Autodesk Inventor part; units mm, degrees
(part 2 of 2)
sketch "Sketch20" plane through (0, 0, 0) normal (0, 0, -1) x (-1, 0, 0)
  circle A0 centre (71.2839, 4.1003) radius 2.05 projected
  line L0 (18.7922, 50.612) -> (16.144, 53.2617) projected
  line L1 (16.144, 53.2617) -> (8.7758, 73.5057) projected
  line L2 (8.7758, 73.5057) -> (-5.3196, 68.3754) projected
  line L3 (-5.3196, 68.3754) -> (-0.5189, 55.1856) projected
  line L4 (-0.5189, 55.1856) -> (-4.7023, 50.8809) projected
  line L5 (-4.7023, 50.8809) -> (-16.3483, 60.653) projected
  line L6 (-16.3483, 60.653) -> (-25.9901, 49.1624) projected
  line L7 (-25.9901, 49.1624) -> (-15.1841, 40.095) projected
  line L8 (-15.1841, 40.095) -> (-24.8028, 30.1972) projected
  line L9 (-24.8028, 30.1972) -> (-34.8028, 30.1972) projected
  line L10 (-34.8028, 30.1972) -> (-34.8028, 10.1972) projected
  line L11 (-34.8028, 10.1972) -> (-29.0502, 10.1972) projected
  arc A1 (-25.3547, 7.7279) -> (-29.0502, 10.1972) centre (-29.0502, 6.1972) ccw projected
  line L12 (-25.3547, 7.7279) -> (-20.83, -3.1958) projected
  arc A2 (-21.6971, -7.5549) -> (-20.83, -3.1958) centre (-24.5255, -4.7265) ccw projected
  line L13 (-21.6971, -7.5549) -> (-25.7648, -11.6226) projected
  line L14 (-25.7648, -11.6226) -> (-11.6226, -25.7648) projected
  line L15 (-11.6226, -25.7648) -> (-7.5549, -21.6971) projected
  arc A3 (-3.1958, -20.83) -> (-7.5549, -21.6971) centre (-4.7265, -24.5255) ccw projected
  line L16 (-3.1958, -20.83) -> (7.7279, -25.3547) projected
  arc A4 (10.1972, -29.0502) -> (7.7279, -25.3547) centre (6.1972, -29.0502) ccw projected
  line L17 (10.1972, -29.0502) -> (10.1972, -34.8028) projected
  line L18 (10.1972, -34.8028) -> (30.1972, -34.8028) projected
  line L19 (30.1972, -34.8028) -> (30.1972, -28.1837) projected
  arc A5 (32.6218, -22.4466) -> (30.1972, -28.1837) centre (38.1972, -28.1837) ccw projected
  line L20 (32.6218, -22.4466) -> (53.0032, -2.6398) projected
  arc A6 (60.0735, -2.7409) -> (53.0032, -2.6398) centre (56.4878, -6.2256) ccw projected
  line L21 (60.0735, -2.7409) -> (62.5248, -5.2633) projected
  line L22 (62.5248, -5.2633) -> (77.9523, 0.8165) projected
  line L23 (77.9523, 0.8165) -> (73.9192, 11.0505) projected
  line L24 (73.9192, 11.0505) -> (50.612, 18.7922) projected
  line L25 (50.612, 18.7922) -> (36.1071, 4.2873) projected
  arc A7 (4.2873, 36.1071) -> (36.1071, 4.2873) centre (20.1972, 20.1972) ccw projected
  line L26 (4.2873, 36.1071) -> (18.7922, 50.612) projected
  circle A8 centre (2.0841, -7.6945) radius 2.075 projected
  circle A9 centre (-7.6945, 2.0841) radius 2.075 projected
  circle A10 centre (14.9946, -12.6504) radius 2.075 projected
  circle A11 centre (-12.6504, 14.9946) radius 2.075 projected
  line L27 (-18.8014, 27.6377) -> (-12.6669, 23.6539) projected
  arc A12 (-12.8482, 20.1946) -> (-12.6669, 23.6539) centre (-13.7562, 21.9766) ccw projected
  line L28 (-12.8482, 20.1946) -> (-19.3655, 16.8739) projected
  arc A13 (-22.272, 18.5798) -> (-19.3655, 16.8739) centre (-20.2735, 18.6559) ccw projected
  arc A14 (-21.8703, 26.245) -> (-22.272, 18.5798) centre (20.1972, 20.1972) ccw projected
  arc A15 (-18.8014, 27.6377) -> (-21.8703, 26.245) centre (-19.8907, 25.9604) ccw projected
  line L29 (-18.4561, 11.1323) -> (-11.2317, 9.988) projected
  arc A16 (-9.9903, 6.754) -> (-11.2317, 9.988) centre (-11.5446, 8.0127) ccw projected
  line L30 (-9.9903, 6.754) -> (-14.5934, 1.0696) projected
  arc A17 (-17.9425, 1.4458) -> (-14.5934, 1.0696) centre (-16.1477, 2.3282) ccw projected
  arc A18 (-20.6932, 8.6117) -> (-17.9425, 1.4458) centre (20.1972, 20.1972) ccw projected
  arc A19 (-18.4561, 11.1323) -> (-20.6932, 8.6117) centre (-18.769, 9.1569) ccw projected
  line L31 (16.8739, -19.3655) -> (20.1946, -12.8482) projected
  arc A20 (23.6539, -12.6669) -> (20.1946, -12.8482) centre (21.9766, -13.7562) ccw projected
  line L32 (23.6539, -12.6669) -> (27.6377, -18.8014) projected
  arc A21 (26.245, -21.8703) -> (27.6377, -18.8014) centre (25.9604, -19.8907) ccw projected
  arc A22 (18.5798, -22.272) -> (26.245, -21.8703) centre (20.1972, 20.1972) ccw projected
  arc A23 (16.8739, -19.3655) -> (18.5798, -22.272) centre (18.6559, -20.2735) ccw projected
  line L33 (1.0696, -14.5934) -> (6.754, -9.9903) projected
  arc A24 (9.988, -11.2317) -> (6.754, -9.9903) centre (8.0127, -11.5446) ccw projected
  line L34 (9.988, -11.2317) -> (11.1323, -18.4561) projected
  arc A25 (8.6117, -20.6932) -> (11.1323, -18.4561) centre (9.1569, -18.769) ccw projected
  arc A26 (1.4458, -17.9425) -> (8.6117, -20.6932) centre (20.1972, 20.1972) ccw projected
  arc A27 (1.0696, -14.5934) -> (1.4458, -17.9425) centre (2.3282, -16.1477) ccw projected
  line L35 (-11.4273, -3.8057) -> (-4.3621, -1.9126) projected
  arc A28 (-1.9126, -4.3621) -> (-4.3621, -1.9126) centre (-3.8444, -3.8444) ccw projected
  line L36 (-1.9126, -4.3621) -> (-3.8057, -11.4273) projected
  arc A29 (-7.0183, -12.4458) -> (-3.8057, -11.4273) centre (-5.7376, -10.9097) ccw projected
  arc A30 (-12.4458, -7.0183) -> (-7.0183, -12.4458) centre (20.1972, 20.1972) ccw projected
  arc A31 (-11.4273, -3.8057) -> (-12.4458, -7.0183) centre (-10.9097, -5.7376) ccw projected
  circle A32 centre (38.4172, 1.8124) radius 1.5 projected
  circle A33 centre (1.8124, 1.8124) radius 1.5 projected
  circle A34 centre (1.8124, 38.4172) radius 1.5 projected
  circle A35 centre (26.1972, -31.0318) radius 1.5 projected
  circle A36 centre (-31.0318, 14.1972) radius 1.5 projected
  circle A37 centre (-31.0318, 26.1972) radius 1.5 projected
  circle A38 centre (14.1972, -31.0318) radius 1.5 projected
  circle A39 centre (-11.7845, -20.2698) radius 1.5 projected
  circle A40 centre (-20.2698, -11.7845) radius 1.5 projected
  circle A41 centre (6.2141, 68.8487) radius 2 projected
  circle A42 centre (-0.3638, 66.4546) radius 2 projected
  circle A43 centre (-18.4881, 52.658) radius 2 projected
  point P0 (0, 0)
hole "Hole4" at (-6.2141, 68.8487, 0) at (0.3638, 66.4546, 0) at (18.4881, 52.658, 0) direction (0, 0, 1) diameter 3 depth 17
fillet "Fillet9" radius 6 1 edges at (24.8028, 30.1972, 2.5)
fillet "Fillet10" radius 3 2 edges at (15.1841, 40.095, 2.5) (4.7023, 50.8809, 2.5)
fillet "Fillet11" radius 4 1 edges at (0.5189, 55.1856, 2.5)
fillet "Fillet12" radius 8 1 edges at (-16.144, 53.2617, 2.5)
sketch "Sketch21" plane through (0, 0, 0) normal (0, 0, -1) x (-1, 0, 0)
  circle A0 centre (-0.3638, 66.4546) radius 1.5 projected
  circle A1 centre (6.2141, 68.8487) radius 1.5 projected
  circle A2 centre (-18.4881, 52.658) radius 1.5 projected
  circle A3 centre (71.2839, 4.1003) radius 2.05 projected
  line L0 (18.7922, 50.612) -> (17.3969, 52.0081) projected
  arc A4 (15.5379, 54.9271) -> (17.3969, 52.0081) centre (23.0554, 57.6633) ccw projected
  line L1 (15.5379, 54.9271) -> (8.7758, 73.5057) projected
  line L2 (8.7758, 73.5057) -> (-5.3196, 68.3754) projected
  line L3 (-5.3196, 68.3754) -> (-1.3768, 57.5426) projected
  arc A5 (-2.267, 53.3868) -> (-1.3768, 57.5426) centre (-5.1356, 56.1745) ccw projected
  line L4 (-2.267, 53.3868) -> (-2.7588, 52.8808) projected
  arc A6 (-6.8386, 52.6734) -> (-2.7588, 52.8808) centre (-4.9102, 54.9716) ccw projected
  line L5 (-6.8386, 52.6734) -> (-16.3483, 60.653) projected
  line L6 (-16.3483, 60.653) -> (-25.9901, 49.1624) projected
  line L7 (-25.9901, 49.1624) -> (-17.6563, 42.1695) projected
  arc A7 (-17.4332, 37.7806) -> (-17.6563, 42.1695) centre (-19.5847, 39.8713) ccw projected
  line L8 (-17.4332, 37.7806) -> (-23.0356, 32.0156) projected
  arc A8 (-27.3385, 30.1972) -> (-23.0356, 32.0156) centre (-27.3385, 36.1972) ccw projected
  line L9 (-27.3385, 30.1972) -> (-34.8028, 30.1972) projected
  line L10 (-34.8028, 30.1972) -> (-34.8028, 10.1972) projected
  line L11 (-34.8028, 10.1972) -> (-29.0502, 10.1972) projected
  arc A9 (-25.3547, 7.7279) -> (-29.0502, 10.1972) centre (-29.0502, 6.1972) ccw projected
  line L12 (-25.3547, 7.7279) -> (-20.83, -3.1958) projected
  arc A10 (-21.6971, -7.5549) -> (-20.83, -3.1958) centre (-24.5255, -4.7265) ccw projected
  line L13 (-21.6971, -7.5549) -> (-25.7648, -11.6226) projected
  line L14 (-25.7648, -11.6226) -> (-11.6226, -25.7648) projected
  line L15 (-11.6226, -25.7648) -> (-7.5549, -21.6971) projected
  arc A11 (-3.1958, -20.83) -> (-7.5549, -21.6971) centre (-4.7265, -24.5255) ccw projected
  line L16 (-3.1958, -20.83) -> (7.7279, -25.3547) projected
  arc A12 (10.1972, -29.0502) -> (7.7279, -25.3547) centre (6.1972, -29.0502) ccw projected
  line L17 (10.1972, -29.0502) -> (10.1972, -34.8028) projected
  line L18 (10.1972, -34.8028) -> (30.1972, -34.8028) projected
  line L19 (30.1972, -34.8028) -> (30.1972, -28.1837) projected
  arc A13 (32.6218, -22.4466) -> (30.1972, -28.1837) centre (38.1972, -28.1837) ccw projected
  line L20 (32.6218, -22.4466) -> (53.0032, -2.6398) projected
  arc A14 (60.0735, -2.7409) -> (53.0032, -2.6398) centre (56.4878, -6.2256) ccw projected
  line L21 (60.0735, -2.7409) -> (62.5248, -5.2633) projected
  line L22 (62.5248, -5.2633) -> (77.9523, 0.8165) projected
  line L23 (77.9523, 0.8165) -> (73.9192, 11.0505) projected
  line L24 (73.9192, 11.0505) -> (50.612, 18.7922) projected
  line L25 (50.612, 18.7922) -> (36.1071, 4.2873) projected
  arc A15 (4.2873, 36.1071) -> (36.1071, 4.2873) centre (20.1972, 20.1972) ccw projected
  line L26 (4.2873, 36.1071) -> (18.7922, 50.612) projected
  circle A16 centre (2.0841, -7.6945) radius 2.075 projected
  circle A17 centre (-7.6945, 2.0841) radius 2.075 projected
  circle A18 centre (14.9946, -12.6504) radius 2.075 projected
  circle A19 centre (-12.6504, 14.9946) radius 2.075 projected
  line L27 (-18.8014, 27.6377) -> (-12.6669, 23.6539) projected
  arc A20 (-12.8482, 20.1946) -> (-12.6669, 23.6539) centre (-13.7562, 21.9766) ccw projected
  line L28 (-12.8482, 20.1946) -> (-19.3655, 16.8739) projected
  arc A21 (-22.272, 18.5798) -> (-19.3655, 16.8739) centre (-20.2735, 18.6559) ccw projected
  arc A22 (-21.8703, 26.245) -> (-22.272, 18.5798) centre (20.1972, 20.1972) ccw projected
  arc A23 (-18.8014, 27.6377) -> (-21.8703, 26.245) centre (-19.8907, 25.9604) ccw projected
  line L29 (-18.4561, 11.1323) -> (-11.2317, 9.988) projected
  arc A24 (-9.9903, 6.754) -> (-11.2317, 9.988) centre (-11.5446, 8.0127) ccw projected
  line L30 (-9.9903, 6.754) -> (-14.5934, 1.0696) projected
  arc A25 (-17.9425, 1.4458) -> (-14.5934, 1.0696) centre (-16.1477, 2.3282) ccw projected
  arc A26 (-20.6932, 8.6117) -> (-17.9425, 1.4458) centre (20.1972, 20.1972) ccw projected
  arc A27 (-18.4561, 11.1323) -> (-20.6932, 8.6117) centre (-18.769, 9.1569) ccw projected
  line L31 (16.8739, -19.3655) -> (20.1946, -12.8482) projected
  arc A28 (23.6539, -12.6669) -> (20.1946, -12.8482) centre (21.9766, -13.7562) ccw projected
  line L32 (23.6539, -12.6669) -> (27.6377, -18.8014) projected
  arc A29 (26.245, -21.8703) -> (27.6377, -18.8014) centre (25.9604, -19.8907) ccw projected
  arc A30 (18.5798, -22.272) -> (26.245, -21.8703) centre (20.1972, 20.1972) ccw projected
  arc A31 (16.8739, -19.3655) -> (18.5798, -22.272) centre (18.6559, -20.2735) ccw projected
  line L33 (1.0696, -14.5934) -> (6.754, -9.9903) projected
  arc A32 (9.988, -11.2317) -> (6.754, -9.9903) centre (8.0127, -11.5446) ccw projected
  line L34 (9.988, -11.2317) -> (11.1323, -18.4561) projected
  arc A33 (8.6117, -20.6932) -> (11.1323, -18.4561) centre (9.1569, -18.769) ccw projected
  arc A34 (1.4458, -17.9425) -> (8.6117, -20.6932) centre (20.1972, 20.1972) ccw projected
  arc A35 (1.0696, -14.5934) -> (1.4458, -17.9425) centre (2.3282, -16.1477) ccw projected
  line L35 (-11.4273, -3.8057) -> (-4.3621, -1.9126) projected
  arc A36 (-1.9126, -4.3621) -> (-4.3621, -1.9126) centre (-3.8444, -3.8444) ccw projected
  line L36 (-1.9126, -4.3621) -> (-3.8057, -11.4273) projected
  arc A37 (-7.0183, -12.4458) -> (-3.8057, -11.4273) centre (-5.7376, -10.9097) ccw projected
  arc A38 (-12.4458, -7.0183) -> (-7.0183, -12.4458) centre (20.1972, 20.1972) ccw projected
  arc A39 (-11.4273, -3.8057) -> (-12.4458, -7.0183) centre (-10.9097, -5.7376) ccw projected
  circle A40 centre (38.4172, 1.8124) radius 1.5 projected
  circle A41 centre (1.8124, 1.8124) radius 1.5 projected
  circle A42 centre (1.8124, 38.4172) radius 1.5 projected
  circle A43 centre (26.1972, -31.0318) radius 1.5 projected
  circle A44 centre (-31.0318, 14.1972) radius 1.5 projected
  circle A45 centre (-31.0318, 26.1972) radius 1.5 projected
  circle A46 centre (14.1972, -31.0318) radius 1.5 projected
  circle A47 centre (-11.7845, -20.2698) radius 1.5 projected
  circle A48 centre (-20.2698, -11.7845) radius 1.5 projected
  line L37 (31.6767, -17.1814) -> (25.3462, -7.4334)
  line L38 (25.3462, -7.4334) -> (41.5924, -1.0919)
  line L39 (41.5924, -1.0919) -> (43.4186, -5.7705)
  line L40 (43.4186, -5.7705) -> (31.6767, -17.1814)
  line L41 (23.6539, -12.6669) -> (27.6377, -18.8014) projected
  line L42 (46.5296, -1.8774) -> (43.6875, 5.5512)
  line L43 (43.6875, 5.5512) -> (51.5169, 13.3805)
  line L44 (51.5169, 13.3805) -> (46.5296, -1.8774)
  line L45 (52.3971, 3.0674) -> (55.3518, 12.1067)
  line L46 (55.3518, 12.1067) -> (66.1951, 8.505)
  line L47 (66.1951, 8.505) -> (52.3971, 3.0674)
  line L48 (55.3518, 12.1067) -> (51.5169, 13.3805)
  line L49 (73.9192, 11.0505) -> (50.612, 18.7922) projected
  line L50 (52.3971, 3.0674) -> (46.5296, -1.8774)
  point P0 (0, 0)
  constraints: 24 end point, 7 parallel, 1 perpendicular
extrude "Extrusion17" cut sketch "Sketch21" against normal blind 5 contours L37 L38 L39 L40 | L42 L43 L44 | L44 L48 L45 L50 | L45 L46 L47
fillet "Fillet16" radius 2 4 edges at (-31.6767, -17.1814, 2.5) (-25.3462, -7.4334, 2.5) (-41.5924, -1.0919, 2.5) (-43.4186, -5.7705, 2.5)
thicken "Thicken2" operation add thickness 1 both sides no extend neighbours yes toward (-0.7071068, -0.7071068, 0) faces at (-48.9071, 10.7708, 1.6667)
thicken "Thicken3" operation add thickness 1 both sides no extend neighbours yes toward (0.3152249, -0.949017, 0) faces at (-57.1174, 11.5203, 3.3333)
fillet "Fillet17" radius 2 1 edges at (-64.7442, 7.9333, 2.5)
fillet "Fillet18" radius 10 1 edges at (-52.3971, 3.0674, 2.5)
fillet "Fillet19" radius 2 1 edges at (-46.5296, -1.8774, 2.5)
fillet "Fillet20" radius 2 2 edges at (-44.0789, 4.5283, 2.5) (-51.7875, 12.2369, 2.5)
sketch "Sketch22" plane through (0, 0, 0) normal (0, 0, -1) x (-1, 0, 0)
  arc A0 (53.9218, 3.6682) -> (51.1441, 2.0113) centre (57.5882, -5.6354) ccw projected
  line L0 (51.1441, 2.0113) -> (48.681, -0.0643) projected
  arc A1 (45.5242, 0.7504) -> (48.681, -0.0643) centre (47.3922, 1.465) ccw projected
  line L1 (45.5242, 0.7504) -> (44.5424, 3.3167) projected
  arc A2 (44.9961, 5.4456) -> (44.5424, 3.3167) centre (46.4104, 4.0313) ccw projected
  line L2 (44.9961, 5.4456) -> (50.9145, 11.3639) projected
  arc A3 (52.9592, 11.8478) -> (50.9145, 11.3639) centre (52.3287, 9.9497) ccw projected
  line L3 (52.9592, 11.8478) -> (59.5128, 9.6709) projected
  arc A4 (59.6157, 5.9121) -> (59.5128, 9.6709) centre (58.8824, 7.7729) ccw projected
  line L4 (59.6157, 5.9121) -> (53.9218, 3.6682) projected
  line L5 (42.3197, -2.955) -> (42.936, -4.534) projected
  arc A5 (42.4668, -6.6955) -> (42.936, -4.534) centre (41.0729, -5.2612) ccw projected
  line L6 (42.4668, -6.6955) -> (33.4222, -15.4851) projected
  arc A6 (30.351, -15.1401) -> (33.4222, -15.4851) centre (32.0283, -14.0508) ccw projected
  line L7 (30.351, -15.1401) -> (26.6837, -9.4929) projected
  arc A7 (27.6338, -6.5405) -> (26.6837, -9.4929) centre (28.361, -8.4036) ccw projected
  line L8 (27.6338, -6.5405) -> (39.7293, -1.8191) projected
  arc A8 (42.3197, -2.955) -> (39.7293, -1.8191) centre (40.4566, -3.6822) ccw projected
  circle A9 centre (-0.3638, 66.4546) radius 1.5 projected
  circle A10 centre (6.2141, 68.8487) radius 1.5 projected
  circle A11 centre (-18.4881, 52.658) radius 1.5 projected
  circle A12 centre (71.2839, 4.1003) radius 2.05 projected
  line L9 (18.7922, 50.612) -> (17.3969, 52.0081) projected
  arc A13 (15.5379, 54.9271) -> (17.3969, 52.0081) centre (23.0554, 57.6633) ccw projected
  line L10 (15.5379, 54.9271) -> (8.7758, 73.5057) projected
  line L11 (8.7758, 73.5057) -> (-5.3196, 68.3754) projected
  line L12 (-5.3196, 68.3754) -> (-1.3768, 57.5426) projected
  arc A14 (-2.267, 53.3868) -> (-1.3768, 57.5426) centre (-5.1356, 56.1745) ccw projected
  line L13 (-2.267, 53.3868) -> (-2.7588, 52.8808) projected
  arc A15 (-6.8386, 52.6734) -> (-2.7588, 52.8808) centre (-4.9102, 54.9716) ccw projected
  line L14 (-6.8386, 52.6734) -> (-16.3483, 60.653) projected
  line L15 (-16.3483, 60.653) -> (-25.9901, 49.1624) projected
  line L16 (-25.9901, 49.1624) -> (-17.6563, 42.1695) projected
  arc A16 (-17.4332, 37.7806) -> (-17.6563, 42.1695) centre (-19.5847, 39.8713) ccw projected
  line L17 (-17.4332, 37.7806) -> (-23.0356, 32.0156) projected
  arc A17 (-27.3385, 30.1972) -> (-23.0356, 32.0156) centre (-27.3385, 36.1972) ccw projected
  line L18 (-27.3385, 30.1972) -> (-34.8028, 30.1972) projected
  line L19 (-34.8028, 30.1972) -> (-34.8028, 10.1972) projected
  line L20 (-34.8028, 10.1972) -> (-29.0502, 10.1972) projected
  arc A18 (-25.3547, 7.7279) -> (-29.0502, 10.1972) centre (-29.0502, 6.1972) ccw projected
  line L21 (-25.3547, 7.7279) -> (-20.83, -3.1958) projected
  arc A19 (-21.6971, -7.5549) -> (-20.83, -3.1958) centre (-24.5255, -4.7265) ccw projected
  line L22 (-21.6971, -7.5549) -> (-25.7648, -11.6226) projected
  line L23 (-25.7648, -11.6226) -> (-11.6226, -25.7648) projected
  line L24 (-11.6226, -25.7648) -> (-7.5549, -21.6971) projected
  arc A20 (-3.1958, -20.83) -> (-7.5549, -21.6971) centre (-4.7265, -24.5255) ccw projected
  line L25 (-3.1958, -20.83) -> (7.7279, -25.3547) projected
  arc A21 (10.1972, -29.0502) -> (7.7279, -25.3547) centre (6.1972, -29.0502) ccw projected
  line L26 (10.1972, -29.0502) -> (10.1972, -34.8028) projected
  line L27 (10.1972, -34.8028) -> (30.1972, -34.8028) projected
  line L28 (30.1972, -34.8028) -> (30.1972, -28.1837) projected
  arc A22 (32.6218, -22.4466) -> (30.1972, -28.1837) centre (38.1972, -28.1837) ccw projected
  line L29 (32.6218, -22.4466) -> (53.0032, -2.6398) projected
  arc A23 (60.0735, -2.7409) -> (53.0032, -2.6398) centre (56.4878, -6.2256) ccw projected
  line L30 (60.0735, -2.7409) -> (62.5248, -5.2633) projected
  line L31 (62.5248, -5.2633) -> (77.9523, 0.8165) projected
  line L32 (77.9523, 0.8165) -> (73.9192, 11.0505) projected
  line L33 (73.9192, 11.0505) -> (50.612, 18.7922) projected
  line L34 (50.612, 18.7922) -> (36.1071, 4.2873) projected
  arc A24 (4.2873, 36.1071) -> (36.1071, 4.2873) centre (20.1972, 20.1972) ccw projected
  line L35 (4.2873, 36.1071) -> (18.7922, 50.612) projected
  circle A25 centre (2.0841, -7.6945) radius 2.075 projected
  circle A26 centre (-7.6945, 2.0841) radius 2.075 projected
  circle A27 centre (14.9946, -12.6504) radius 2.075 projected
  circle A28 centre (-12.6504, 14.9946) radius 2.075 projected
  line L36 (-18.8014, 27.6377) -> (-12.6669, 23.6539) projected
  arc A29 (-12.8482, 20.1946) -> (-12.6669, 23.6539) centre (-13.7562, 21.9766) ccw projected
  line L37 (-12.8482, 20.1946) -> (-19.3655, 16.8739) projected
  arc A30 (-22.272, 18.5798) -> (-19.3655, 16.8739) centre (-20.2735, 18.6559) ccw projected
  arc A31 (-21.8703, 26.245) -> (-22.272, 18.5798) centre (20.1972, 20.1972) ccw projected
  arc A32 (-18.8014, 27.6377) -> (-21.8703, 26.245) centre (-19.8907, 25.9604) ccw projected
  line L38 (-18.4561, 11.1323) -> (-11.2317, 9.988) projected
  arc A33 (-9.9903, 6.754) -> (-11.2317, 9.988) centre (-11.5446, 8.0127) ccw projected
  line L39 (-9.9903, 6.754) -> (-14.5934, 1.0696) projected
  arc A34 (-17.9425, 1.4458) -> (-14.5934, 1.0696) centre (-16.1477, 2.3282) ccw projected
  arc A35 (-20.6932, 8.6117) -> (-17.9425, 1.4458) centre (20.1972, 20.1972) ccw projected
  arc A36 (-18.4561, 11.1323) -> (-20.6932, 8.6117) centre (-18.769, 9.1569) ccw projected
  line L40 (16.8739, -19.3655) -> (20.1946, -12.8482) projected
  arc A37 (23.6539, -12.6669) -> (20.1946, -12.8482) centre (21.9766, -13.7562) ccw projected
  line L41 (23.6539, -12.6669) -> (27.6377, -18.8014) projected
  arc A38 (26.245, -21.8703) -> (27.6377, -18.8014) centre (25.9604, -19.8907) ccw projected
  arc A39 (18.5798, -22.272) -> (26.245, -21.8703) centre (20.1972, 20.1972) ccw projected
  arc A40 (16.8739, -19.3655) -> (18.5798, -22.272) centre (18.6559, -20.2735) ccw projected
  line L42 (1.0696, -14.5934) -> (6.754, -9.9903) projected
  arc A41 (9.988, -11.2317) -> (6.754, -9.9903) centre (8.0127, -11.5446) ccw projected
  line L43 (9.988, -11.2317) -> (11.1323, -18.4561) projected
  arc A42 (8.6117, -20.6932) -> (11.1323, -18.4561) centre (9.1569, -18.769) ccw projected
  arc A43 (1.4458, -17.9425) -> (8.6117, -20.6932) centre (20.1972, 20.1972) ccw projected
  arc A44 (1.0696, -14.5934) -> (1.4458, -17.9425) centre (2.3282, -16.1477) ccw projected
  line L44 (-11.4273, -3.8057) -> (-4.3621, -1.9126) projected
  arc A45 (-1.9126, -4.3621) -> (-4.3621, -1.9126) centre (-3.8444, -3.8444) ccw projected
  line L45 (-1.9126, -4.3621) -> (-3.8057, -11.4273) projected
  arc A46 (-7.0183, -12.4458) -> (-3.8057, -11.4273) centre (-5.7376, -10.9097) ccw projected
  arc A47 (-12.4458, -7.0183) -> (-7.0183, -12.4458) centre (20.1972, 20.1972) ccw projected
  arc A48 (-11.4273, -3.8057) -> (-12.4458, -7.0183) centre (-10.9097, -5.7376) ccw projected
  circle A49 centre (38.4172, 1.8124) radius 1.5 projected
  circle A50 centre (1.8124, 1.8124) radius 1.5 projected
  circle A51 centre (1.8124, 38.4172) radius 1.5 projected
  circle A52 centre (26.1972, -31.0318) radius 1.5 projected
  circle A53 centre (-31.0318, 14.1972) radius 1.5 projected
  circle A54 centre (-31.0318, 26.1972) radius 1.5 projected
  circle A55 centre (14.1972, -31.0318) radius 1.5 projected
  circle A56 centre (-11.7845, -20.2698) radius 1.5 projected
  circle A57 centre (-20.2698, -11.7845) radius 1.5 projected
  circle A58 centre (-0.3638, 66.4546) radius 1.5 projected
  circle A59 centre (6.2141, 68.8487) radius 1.5 projected
  line L46 (-0.3638, 66.4546) -> (6.2141, 68.8487)
  line L47 (2.9252, 67.6517) -> (7.0294, 56.3753)
  circle A60 centre (-18.4881, 52.658) radius 1.5 projected
  line L48 (-18.4881, 52.658) -> (-9.2955, 44.9445)
  line L49 (-6.8386, 52.6734) -> (-16.3483, 60.653) projected
  line L50 (-6.2314, 42.3734) -> (-12.3597, 47.5157) construction
  line L51 (-3.6602, 45.4375) -> (-9.7886, 50.5798)
  line L52 (-14.9309, 44.4515) -> (-8.8025, 39.3092)
  arc A61 (-8.8025, 39.3092) -> (-3.6602, 45.4375) centre (-6.2314, 42.3734) ccw
  arc A62 (-9.7886, 50.5798) -> (-14.9309, 44.4515) centre (-12.3597, 47.5157) ccw
  line L53 (8.3975, 52.6166) -> (5.6613, 60.1341) construction
  line L54 (12.1563, 53.9847) -> (9.4201, 61.5022)
  line L55 (1.9026, 58.766) -> (4.6387, 51.2485)
  arc A63 (4.6387, 51.2485) -> (12.1563, 53.9847) centre (8.3975, 52.6166) ccw
  arc A64 (9.4201, 61.5022) -> (1.9026, 58.766) centre (5.6613, 60.1341) ccw
  point P0 (0, 0)
  dimension "d126" = 12
  dimension "d127" = 12
  dimension "d128" = 4
  dimension "d129" = 8
  dimension "d130" = 4
  dimension "d131" = 8
  constraints: 22 end point, 8 point on circle, 8 tangent, 4 centre point, 3 midpoint, 3 parallel, 2 point on line, 1 perpendicular
  measures "d126" distance of L47.start L47.end
  measures "d127" distance of L48.start L48.end
  measures "d128" distance of L48.end L50.end
  measures "d129" diameter of A62
  measures "d130" distance of L47.end L53.end
  measures "d131" diameter of A64
extrude "Extrusion18" cut sketch "Sketch22" against normal blind 5 contours A61 L52 A62 L51 | A63 L55 A64 L54
thicken "Thicken4" operation add thickness 0.5 both sides no extend neighbours yes toward (-0.9396926, 0.3420201, 0) faces at (-2.8146, 56.2602, 1.6667)
thicken "Thicken5" operation add thickness 0.5 both sides no extend neighbours yes toward (-0.6427876, 0.7660444, 0) faces at (10.8453, 41.0233, 3.3333)
sketch "Sketch23" plane through (0, 0, 0) normal (0, 0, -1) x (-1, 0, 0)
  line L0 (5.1086, 51.4195) -> (2.3724, 58.937) projected
  arc A0 (8.9502, 61.3312) -> (2.3724, 58.937) centre (5.6613, 60.1341) ccw projected
  line L1 (8.9502, 61.3312) -> (11.6864, 53.8136) projected
  arc A1 (5.1086, 51.4195) -> (11.6864, 53.8136) centre (8.3975, 52.6166) ccw projected
  line L2 (-8.4811, 39.6922) -> (-14.6095, 44.8345) projected
  arc A2 (-10.11, 50.1968) -> (-14.6095, 44.8345) centre (-12.3597, 47.5157) ccw projected
  line L3 (-10.11, 50.1968) -> (-3.9816, 45.0545) projected
  arc A3 (-8.4811, 39.6922) -> (-3.9816, 45.0545) centre (-6.2314, 42.3734) ccw projected
  arc A4 (53.9218, 3.6682) -> (51.1441, 2.0113) centre (57.5882, -5.6354) ccw projected
  line L4 (51.1441, 2.0113) -> (48.681, -0.0643) projected
  arc A5 (45.5242, 0.7504) -> (48.681, -0.0643) centre (47.3922, 1.465) ccw projected
  line L5 (45.5242, 0.7504) -> (44.5424, 3.3167) projected
  arc A6 (44.9961, 5.4456) -> (44.5424, 3.3167) centre (46.4104, 4.0313) ccw projected
  line L6 (44.9961, 5.4456) -> (50.9145, 11.3639) projected
  arc A7 (52.9592, 11.8478) -> (50.9145, 11.3639) centre (52.3287, 9.9497) ccw projected
  line L7 (52.9592, 11.8478) -> (59.5128, 9.6709) projected
  arc A8 (59.6157, 5.9121) -> (59.5128, 9.6709) centre (58.8824, 7.7729) ccw projected
  line L8 (59.6157, 5.9121) -> (53.9218, 3.6682) projected
  line L9 (42.3197, -2.955) -> (42.936, -4.534) projected
  arc A9 (42.4668, -6.6955) -> (42.936, -4.534) centre (41.0729, -5.2612) ccw projected
  line L10 (42.4668, -6.6955) -> (33.4222, -15.4851) projected
  arc A10 (30.351, -15.1401) -> (33.4222, -15.4851) centre (32.0283, -14.0508) ccw projected
  line L11 (30.351, -15.1401) -> (26.6837, -9.4929) projected
  arc A11 (27.6338, -6.5405) -> (26.6837, -9.4929) centre (28.361, -8.4036) ccw projected
  line L12 (27.6338, -6.5405) -> (39.7293, -1.8191) projected
  arc A12 (42.3197, -2.955) -> (39.7293, -1.8191) centre (40.4566, -3.6822) ccw projected
  circle A13 centre (-0.3638, 66.4546) radius 1.5 projected
  circle A14 centre (6.2141, 68.8487) radius 1.5 projected
  circle A15 centre (-18.4881, 52.658) radius 1.5 projected
  circle A16 centre (71.2839, 4.1003) radius 2.05 projected
  line L13 (18.7922, 50.612) -> (17.3969, 52.0081) projected
  arc A17 (15.5379, 54.9271) -> (17.3969, 52.0081) centre (23.0554, 57.6633) ccw projected
  line L14 (15.5379, 54.9271) -> (8.7758, 73.5057) projected
  line L15 (8.7758, 73.5057) -> (-5.3196, 68.3754) projected
  line L16 (-5.3196, 68.3754) -> (-1.3768, 57.5426) projected
  arc A18 (-2.267, 53.3868) -> (-1.3768, 57.5426) centre (-5.1356, 56.1745) ccw projected
  line L17 (-2.267, 53.3868) -> (-2.7588, 52.8808) projected
  arc A19 (-6.8386, 52.6734) -> (-2.7588, 52.8808) centre (-4.9102, 54.9716) ccw projected
  line L18 (-6.8386, 52.6734) -> (-16.3483, 60.653) projected
  line L19 (-16.3483, 60.653) -> (-25.9901, 49.1624) projected
  line L20 (-25.9901, 49.1624) -> (-17.6563, 42.1695) projected
  arc A20 (-17.4332, 37.7806) -> (-17.6563, 42.1695) centre (-19.5847, 39.8713) ccw projected
  line L21 (-17.4332, 37.7806) -> (-23.0356, 32.0156) projected
  arc A21 (-27.3385, 30.1972) -> (-23.0356, 32.0156) centre (-27.3385, 36.1972) ccw projected
  line L22 (-27.3385, 30.1972) -> (-34.8028, 30.1972) projected
  line L23 (-34.8028, 30.1972) -> (-34.8028, 10.1972) projected
  line L24 (-34.8028, 10.1972) -> (-29.0502, 10.1972) projected
  arc A22 (-25.3547, 7.7279) -> (-29.0502, 10.1972) centre (-29.0502, 6.1972) ccw projected
  line L25 (-25.3547, 7.7279) -> (-20.83, -3.1958) projected
  arc A23 (-21.6971, -7.5549) -> (-20.83, -3.1958) centre (-24.5255, -4.7265) ccw projected
  line L26 (-21.6971, -7.5549) -> (-25.7648, -11.6226) projected
  line L27 (-25.7648, -11.6226) -> (-11.6226, -25.7648) projected
  line L28 (-11.6226, -25.7648) -> (-7.5549, -21.6971) projected
  arc A24 (-3.1958, -20.83) -> (-7.5549, -21.6971) centre (-4.7265, -24.5255) ccw projected
  line L29 (-3.1958, -20.83) -> (7.7279, -25.3547) projected
  arc A25 (10.1972, -29.0502) -> (7.7279, -25.3547) centre (6.1972, -29.0502) ccw projected
  line L30 (10.1972, -29.0502) -> (10.1972, -34.8028) projected
  line L31 (10.1972, -34.8028) -> (30.1972, -34.8028) projected
  line L32 (30.1972, -34.8028) -> (30.1972, -28.1837) projected
  arc A26 (32.6218, -22.4466) -> (30.1972, -28.1837) centre (38.1972, -28.1837) ccw projected
  line L33 (32.6218, -22.4466) -> (53.0032, -2.6398) projected
  arc A27 (60.0735, -2.7409) -> (53.0032, -2.6398) centre (56.4878, -6.2256) ccw projected
  line L34 (60.0735, -2.7409) -> (62.5248, -5.2633) projected
  line L35 (62.5248, -5.2633) -> (77.9523, 0.8165) projected
  line L36 (77.9523, 0.8165) -> (73.9192, 11.0505) projected
  line L37 (73.9192, 11.0505) -> (50.612, 18.7922) projected
  line L38 (50.612, 18.7922) -> (36.1071, 4.2873) projected
  arc A28 (4.2873, 36.1071) -> (36.1071, 4.2873) centre (20.1972, 20.1972) ccw projected
  line L39 (4.2873, 36.1071) -> (18.7922, 50.612) projected
  circle A29 centre (2.0841, -7.6945) radius 2.075 projected
  circle A30 centre (-7.6945, 2.0841) radius 2.075 projected
  circle A31 centre (14.9946, -12.6504) radius 2.075 projected
  circle A32 centre (-12.6504, 14.9946) radius 2.075 projected
  line L40 (-18.8014, 27.6377) -> (-12.6669, 23.6539) projected
  arc A33 (-12.8482, 20.1946) -> (-12.6669, 23.6539) centre (-13.7562, 21.9766) ccw projected
  line L41 (-12.8482, 20.1946) -> (-19.3655, 16.8739) projected
  arc A34 (-22.272, 18.5798) -> (-19.3655, 16.8739) centre (-20.2735, 18.6559) ccw projected
  arc A35 (-21.8703, 26.245) -> (-22.272, 18.5798) centre (20.1972, 20.1972) ccw projected
  arc A36 (-18.8014, 27.6377) -> (-21.8703, 26.245) centre (-19.8907, 25.9604) ccw projected
  line L42 (-18.4561, 11.1323) -> (-11.2317, 9.988) projected
  arc A37 (-9.9903, 6.754) -> (-11.2317, 9.988) centre (-11.5446, 8.0127) ccw projected
  line L43 (-9.9903, 6.754) -> (-14.5934, 1.0696) projected
  arc A38 (-17.9425, 1.4458) -> (-14.5934, 1.0696) centre (-16.1477, 2.3282) ccw projected
  arc A39 (-20.6932, 8.6117) -> (-17.9425, 1.4458) centre (20.1972, 20.1972) ccw projected
  arc A40 (-18.4561, 11.1323) -> (-20.6932, 8.6117) centre (-18.769, 9.1569) ccw projected
  line L44 (16.8739, -19.3655) -> (20.1946, -12.8482) projected
  arc A41 (23.6539, -12.6669) -> (20.1946, -12.8482) centre (21.9766, -13.7562) ccw projected
  line L45 (23.6539, -12.6669) -> (27.6377, -18.8014) projected
  arc A42 (26.245, -21.8703) -> (27.6377, -18.8014) centre (25.9604, -19.8907) ccw projected
  arc A43 (18.5798, -22.272) -> (26.245, -21.8703) centre (20.1972, 20.1972) ccw projected
  arc A44 (16.8739, -19.3655) -> (18.5798, -22.272) centre (18.6559, -20.2735) ccw projected
  line L46 (1.0696, -14.5934) -> (6.754, -9.9903) projected
  arc A45 (9.988, -11.2317) -> (6.754, -9.9903) centre (8.0127, -11.5446) ccw projected
  line L47 (9.988, -11.2317) -> (11.1323, -18.4561) projected
  arc A46 (8.6117, -20.6932) -> (11.1323, -18.4561) centre (9.1569, -18.769) ccw projected
  arc A47 (1.4458, -17.9425) -> (8.6117, -20.6932) centre (20.1972, 20.1972) ccw projected
  arc A48 (1.0696, -14.5934) -> (1.4458, -17.9425) centre (2.3282, -16.1477) ccw projected
  line L48 (-11.4273, -3.8057) -> (-4.3621, -1.9126) projected
  arc A49 (-1.9126, -4.3621) -> (-4.3621, -1.9126) centre (-3.8444, -3.8444) ccw projected
  line L49 (-1.9126, -4.3621) -> (-3.8057, -11.4273) projected
  arc A50 (-7.0183, -12.4458) -> (-3.8057, -11.4273) centre (-5.7376, -10.9097) ccw projected
  arc A51 (-12.4458, -7.0183) -> (-7.0183, -12.4458) centre (20.1972, 20.1972) ccw projected
  arc A52 (-11.4273, -3.8057) -> (-12.4458, -7.0183) centre (-10.9097, -5.7376) ccw projected
  circle A53 centre (38.4172, 1.8124) radius 1.5 projected
  circle A54 centre (1.8124, 1.8124) radius 1.5 projected
  circle A55 centre (1.8124, 38.4172) radius 1.5 projected
  circle A56 centre (26.1972, -31.0318) radius 1.5 projected
  circle A57 centre (-31.0318, 14.1972) radius 1.5 projected
  circle A58 centre (-31.0318, 26.1972) radius 1.5 projected
  circle A59 centre (14.1972, -31.0318) radius 1.5 projected
  circle A60 centre (-11.7845, -20.2698) radius 1.5 projected
  circle A61 centre (-20.2698, -11.7845) radius 1.5 projected
  line L50 (-17.2246, 31.5471) -> (-11.5303, 37.4066)
  line L51 (-11.5303, 37.4066) -> (-4.6245, 31.612)
  line L52 (-4.6245, 31.612) -> (-9.104, 26.2735)
  line L53 (-9.104, 26.2735) -> (-17.2246, 31.5471)
  line L54 (-8.4811, 39.6922) -> (-14.6095, 44.8345) projected
  line L55 (-18.8014, 27.6377) -> (-12.6669, 23.6539) projected
  point P0 (0, 0)
  constraints: 8 end point, 3 parallel, 1 perpendicular
extrude "Extrusion19" cut sketch "Sketch23" against normal blind 5 contours L50 L51 L52 L53
fillet "Fillet21" radius 2 4 edges at (9.104, 26.2735, 2.5) (17.2246, 31.5471, 2.5) (11.5303, 37.4066, 2.5) (4.6245, 31.612, 2.5)
body "Solid1"
